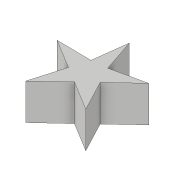
# Autodesk Inventor part: star
Saved by Autodesk Inventor 2019 (Build 230136000, 136)
## iProperties
Created: 2020-06-22
Part Number: star
Material: Generic
Document SubType Name: Modeling
Designer: dmulr
Density: 1 g/cm^3
Appearance: Default
Author: dmulr
Autodesk Inventor part; units mm, degrees
ref_plane "YZ Plane" through (0, 0, 0) normal (1, 0, 0) x (0, 1, 0)
ref_plane "XZ Plane" through (0, 0, 0) normal (0, 1, 0) x (-1, 0, 0)
ref_plane "XY Plane" through (0, 0, 0) normal (0, 0, 1) x (1, 0, 0)
sketch "Sketch1" plane through (0, 0, 0) normal (0, 1, 0) x (-1, 0, 0)
  line L0 (144.1124, -41.6125) -> (46.6139, 18.087)
  line L1 (46.6139, 18.087) -> (78.3294, 127.9238)
  line L2 (78.3294, 127.9238) -> (-5.082, 49.7411)
  line L3 (-5.082, 49.7411) -> (-102.5805, 109.4406)
  line L4 (-102.5805, 109.4406) -> (-49.3085, 8.2868)
  line L5 (-49.3085, 8.2868) -> (-132.7198, -69.896)
  line L6 (-132.7198, -69.896) -> (-21.0625, -45.3472)
  line L7 (-21.0625, -45.3472) -> (15.6932, -153.6016)
  line L8 (15.6932, -153.6016) -> (29.7977, -40.1509)
  line L9 (29.7977, -40.1509) -> (144.1124, -41.6125)
  point P0 (0, 0)
  dimension "d1" = 150
  constraints: 20 end point, 9 equal length, 1 collinear
  measures "d1" distance of point (0, 0) L0.start
extrude "Extrusion1" add sketch "Sketch1" along normal blind 120
body "Solid1"
